Autodesk Fusion 360 part; units mm, degrees
(part 2 of 2)
sketch "Sketch4 (2)" plane through (0, -8, 0) normal (0, 1, 0) x (-1, 0, 0) in component "Middle_Cover"
  arc A0 (-84, -10) -> (-90, -16) centre (-84, -16) ccw
  line L0 (-90, -16) -> (-90, -28)
  arc A1 (-90, -28) -> (-84, -34) centre (-84, -28) ccw
  line L1 (-84, -34) -> (-16, -34)
  arc A2 (-16, -34) -> (-10, -28) centre (-16, -28) ccw
  line L2 (-10, -28) -> (-10, -16)
  arc A3 (-10, -16) -> (-16, -10) centre (-16, -16) ccw
  line L3 (-16, -10) -> (-84, -10)
  line L4 (-50, -22) -> (-90, -22) construction
  line L5 (-80, -12) -> (-60, -12) construction
  line L6 (-60, -12) -> (-60, -32) construction
  line L7 (-60, -32) -> (-80, -32) construction
  line L8 (-80, -32) -> (-80, -12) construction
  line L9 (-80, -12) -> (-60, -32) construction
  line L10 (-60, -12) -> (-80, -32) construction
  line L11 (-80, -32) -> (-60, -32) construction
  line L12 (-60, -32) -> (-60, -30) construction
  line L13 (-60, -30) -> (-80, -30) construction
  line L14 (-80, -30) -> (-80, -32) construction
  line L15 (-60, -30) -> (-80, -30) construction
  line L16 (-80, -30) -> (-80, -28) construction
  line L17 (-80, -28) -> (-60, -28) construction
  line L18 (-60, -28) -> (-60, -30) construction
  line L19 (-60, -28) -> (-80, -28) construction
  line L20 (-80, -28) -> (-80, -26) construction
  line L21 (-80, -26) -> (-60, -26) construction
  line L22 (-60, -26) -> (-60, -28) construction
  line L23 (-60, -26) -> (-80, -26) construction
  line L24 (-80, -26) -> (-80, -24) construction
  line L25 (-80, -24) -> (-60, -24) construction
  line L26 (-60, -24) -> (-60, -26) construction
  line L27 (-60, -22) -> (-80, -22) construction
  line L28 (-80, -22) -> (-80, -24) construction
  line L29 (-80, -24) -> (-60, -24) construction
  line L30 (-60, -24) -> (-60, -22) construction
  line L31 (-60, -22) -> (-80, -22) construction
  line L32 (-80, -22) -> (-80, -20) construction
  line L33 (-80, -20) -> (-60, -20) construction
  line L34 (-60, -20) -> (-60, -22) construction
  line L35 (-60, -20) -> (-80, -20) construction
  line L36 (-80, -20) -> (-80, -18) construction
  line L37 (-80, -18) -> (-60, -18) construction
  line L38 (-60, -18) -> (-60, -20) construction
  line L39 (-60, -18) -> (-80, -18) construction
  line L40 (-80, -18) -> (-80, -16) construction
  line L41 (-80, -16) -> (-60, -16) construction
  line L42 (-60, -16) -> (-60, -18) construction
  line L43 (-60, -16) -> (-80, -16) construction
  line L44 (-80, -16) -> (-80, -14) construction
  line L45 (-80, -14) -> (-60, -14) construction
  line L46 (-60, -14) -> (-60, -16) construction
  line L47 (-80, -12) -> (-78, -12) construction
  line L48 (-78, -12) -> (-78, -32) construction
  line L49 (-78, -32) -> (-80, -32) construction
  line L50 (-80, -32) -> (-80, -12) construction
  line L51 (-78, -32) -> (-76, -32) construction
  line L52 (-76, -32) -> (-76, -12) construction
  line L53 (-76, -12) -> (-78, -12) construction
  line L54 (-78, -12) -> (-78, -32) construction
  line L55 (-76, -32) -> (-74, -32) construction
  line L56 (-74, -32) -> (-74, -12) construction
  line L57 (-74, -12) -> (-76, -12) construction
  line L58 (-76, -12) -> (-76, -32) construction
  line L59 (-74, -32) -> (-72, -32) construction
  line L60 (-72, -32) -> (-72, -12) construction
  line L61 (-72, -12) -> (-74, -12) construction
  line L62 (-74, -12) -> (-74, -32) construction
  line L63 (-72, -32) -> (-70, -32) construction
  line L64 (-70, -32) -> (-70, -12) construction
  line L65 (-70, -12) -> (-72, -12) construction
  line L66 (-72, -12) -> (-72, -32) construction
  line L67 (-70, -12) -> (-68, -12) construction
  line L68 (-68, -12) -> (-68, -32) construction
  line L69 (-68, -32) -> (-70, -32) construction
  line L70 (-70, -32) -> (-70, -12) construction
  line L71 (-68, -32) -> (-66, -32) construction
  line L72 (-66, -32) -> (-66, -12) construction
  line L73 (-66, -12) -> (-68, -12) construction
  line L74 (-68, -12) -> (-68, -32) construction
  line L75 (-66, -32) -> (-64, -32) construction
  line L76 (-64, -32) -> (-64, -12) construction
  line L77 (-64, -12) -> (-66, -12) construction
  line L78 (-66, -12) -> (-66, -32) construction
  line L79 (-64, -32) -> (-62, -32) construction
  line L80 (-62, -32) -> (-62, -12) construction
  line L81 (-62, -12) -> (-64, -12) construction
  line L82 (-64, -12) -> (-64, -32) construction
  circle A4 centre (-78, -30) radius 1.5
  circle A5 centre (-78, -26) radius 1.5
  circle A6 centre (-78, -22) radius 1.5
  circle A7 centre (-78, -18) radius 1.5
  circle A8 centre (-78, -14) radius 1.5
  circle A9 centre (-74, -14) radius 1.5
  circle A10 centre (-74, -18) radius 1.5
  circle A11 centre (-74, -22) radius 1.5
  circle A12 centre (-74, -26) radius 1.5
  circle A13 centre (-74, -30) radius 1.5
  circle A14 centre (-70, -30) radius 1.5
  circle A15 centre (-70, -26) radius 1.5
  circle A16 centre (-70, -22) radius 1.5
  circle A17 centre (-70, -18) radius 1.5
  circle A18 centre (-70, -14) radius 1.5
  circle A19 centre (-66, -14) radius 1.5
  circle A20 centre (-66, -18) radius 1.5
  circle A21 centre (-66, -22) radius 1.5
  circle A22 centre (-66, -26) radius 1.5
  circle A23 centre (-66, -30) radius 1.5
  circle A24 centre (-62, -30) radius 1.5
  circle A25 centre (-62, -26) radius 1.5
  circle A26 centre (-62, -22) radius 1.5
  circle A27 centre (-62, -18) radius 1.5
  circle A28 centre (-62, -14) radius 1.5
  line L83 (-50, -22) -> (-10, -22) construction
  line L84 (-40, -12) -> (-20, -12) construction
  line L85 (-20, -12) -> (-20, -32) construction
  line L86 (-20, -32) -> (-40, -32) construction
  line L87 (-40, -32) -> (-40, -12) construction
  line L88 (-40, -12) -> (-20, -32) construction
  line L89 (-20, -12) -> (-40, -32) construction
  line L90 (-20, -12) -> (-22, -12) construction
  line L91 (-22, -12) -> (-22, -32) construction
  line L92 (-22, -32) -> (-20, -32) construction
  line L93 (-20, -32) -> (-20, -12) construction
  line L94 (-22, -32) -> (-24, -32) construction
  line L95 (-24, -32) -> (-24, -12) construction
  line L96 (-24, -12) -> (-22, -12) construction
  line L97 (-22, -12) -> (-22, -32) construction
  line L98 (-24, -12) -> (-26, -12) construction
  line L99 (-26, -12) -> (-26, -32) construction
  line L100 (-26, -32) -> (-24, -32) construction
  line L101 (-24, -32) -> (-24, -12) construction
  line L102 (-26, -32) -> (-28, -32) construction
  line L103 (-28, -32) -> (-28, -12) construction
  line L104 (-28, -12) -> (-26, -12) construction
  line L105 (-26, -12) -> (-26, -32) construction
  line L106 (-28, -12) -> (-30, -12) construction
  line L107 (-30, -12) -> (-30, -32) construction
  line L108 (-30, -32) -> (-28, -32) construction
  line L109 (-28, -32) -> (-28, -12) construction
  line L110 (-30, -32) -> (-32, -32) construction
  line L111 (-32, -32) -> (-32, -12) construction
  line L112 (-32, -12) -> (-30, -12) construction
  line L113 (-30, -12) -> (-30, -32) construction
  line L114 (-32, -12) -> (-34, -12) construction
  line L115 (-34, -12) -> (-34, -32) construction
  line L116 (-34, -32) -> (-32, -32) construction
  line L117 (-32, -32) -> (-32, -12) construction
  line L118 (-34, -32) -> (-36, -32) construction
  line L119 (-36, -32) -> (-36, -12) construction
  line L120 (-36, -12) -> (-34, -12) construction
  line L121 (-34, -12) -> (-34, -32) construction
  line L122 (-36, -12) -> (-38, -12) construction
  line L123 (-38, -12) -> (-38, -32) construction
  line L124 (-38, -32) -> (-36, -32) construction
  line L125 (-36, -32) -> (-36, -12) construction
  line L126 (-40, -12) -> (-20, -12) construction
  line L127 (-20, -12) -> (-20, -14) construction
  line L128 (-20, -14) -> (-40, -14) construction
  line L129 (-40, -14) -> (-40, -12) construction
  line L130 (-20, -14) -> (-40, -14) construction
  line L131 (-40, -14) -> (-40, -16) construction
  line L132 (-40, -16) -> (-20, -16) construction
  line L133 (-20, -16) -> (-20, -14) construction
  line L134 (-20, -16) -> (-40, -16) construction
  line L135 (-40, -16) -> (-40, -18) construction
  line L136 (-40, -18) -> (-20, -18) construction
  line L137 (-20, -18) -> (-20, -16) construction
  line L138 (-40, -18) -> (-20, -18) construction
  line L139 (-20, -18) -> (-20, -20) construction
  line L140 (-20, -20) -> (-40, -20) construction
  line L141 (-40, -20) -> (-40, -18) construction
  line L142 (-40, -22) -> (-20, -22) construction
  line L143 (-20, -22) -> (-20, -24) construction
  line L144 (-20, -24) -> (-40, -24) construction
  line L145 (-40, -24) -> (-40, -22) construction
  line L146 (-40, -24) -> (-20, -24) construction
  line L147 (-20, -24) -> (-20, -26) construction
  line L148 (-20, -26) -> (-40, -26) construction
  line L149 (-40, -26) -> (-40, -24) construction
  line L150 (-40, -26) -> (-20, -26) construction
  line L151 (-20, -26) -> (-20, -28) construction
  line L152 (-20, -28) -> (-40, -28) construction
  line L153 (-40, -28) -> (-40, -26) construction
  line L154 (-40, -28) -> (-20, -28) construction
  line L155 (-20, -28) -> (-20, -30) construction
  line L156 (-20, -30) -> (-40, -30) construction
  line L157 (-40, -30) -> (-40, -28) construction
  circle A29 centre (-38, -30) radius 1.5
  circle A30 centre (-38, -26) radius 1.5
  circle A31 centre (-38, -22) radius 1.5
  circle A32 centre (-38, -18) radius 1.5
  circle A33 centre (-38, -14) radius 1.5
  circle A34 centre (-34, -14) radius 1.5
  circle A35 centre (-34, -18) radius 1.5
  circle A36 centre (-34, -22) radius 1.5
  circle A37 centre (-34, -26) radius 1.5
  circle A38 centre (-34, -30) radius 1.5
  circle A39 centre (-30, -30) radius 1.5
  circle A40 centre (-30, -26) radius 1.5
  circle A41 centre (-30, -22) radius 1.5
  circle A42 centre (-30, -18) radius 1.5
  circle A43 centre (-30, -14) radius 1.5
  circle A44 centre (-26, -14) radius 1.5
  circle A45 centre (-22, -14) radius 1.5
  circle A46 centre (-26, -18) radius 1.5
  circle A47 centre (-22, -18) radius 1.5
  circle A48 centre (-26, -22) radius 1.5
  circle A49 centre (-22, -22) radius 1.5
  circle A50 centre (-26, -26) radius 1.5
  circle A51 centre (-22, -26) radius 1.5
  circle A52 centre (-22, -30) radius 1.5
  circle A53 centre (-26, -30) radius 1.5
  point P0 (-70, -22)
  point P1 (-30, -22)
  dimension "d20_1" = 20
  dimension "d21_1" = 20
  dimension "d22_1" = 2
  dimension "d23_1" = 2
  dimension "d24_1" = 2
  dimension "d25_1" = 2
  dimension "d26_1" = 2
  dimension "d27_1" = 2
  dimension "d28_1" = 2
  dimension "d29_1" = 2
  dimension "d30_1" = 2
  dimension "d31_1" = 2
  dimension "d32_1" = 2
  dimension "d33_1" = 2
  dimension "d34_1" = 2
  dimension "d35_1" = 3
  dimension "d36_1" = 3
  dimension "d37_1" = 3
  dimension "d38_1" = 3
  dimension "d39_1" = 3
  dimension "d40_1" = 3
  dimension "d41_1" = 3
  dimension "d42_1" = 3
  dimension "d43_1" = 3
  dimension "d44_1" = 3
  dimension "d45_1" = 3
  dimension "d46_1" = 3
  dimension "d47_1" = 3
  dimension "d48_1" = 3
  dimension "d49_1" = 3
  dimension "d50_1" = 3
  dimension "d51_1" = 3
  dimension "d52_1" = 3
  dimension "d53_1" = 3
  dimension "d54_1" = 3
  dimension "d55_1" = 3
  dimension "d56_1" = 3
  dimension "d57_1" = 3
  dimension "d58_1" = 3
  dimension "d59_1" = 3
  dimension "d62_1" = 20
  dimension "d63_1" = 20
  dimension "d64_1" = 2
  dimension "d65_1" = 20
  dimension "d66_1" = 2
  dimension "d67_1" = 2
  dimension "d68_1" = 2
  dimension "d69_1" = 2
  dimension "d70_1" = 2
  dimension "d71_1" = 20
  dimension "d72_1" = 2
  dimension "d73_1" = 2
  dimension "d74_1" = 2
  dimension "d75_1" = 2
  dimension "d76_1" = 2
  dimension "d77_1" = 2
  dimension "d78_1" = 3
  dimension "d79_1" = 3
  dimension "d80_1" = 3
  dimension "d81_1" = 3
  dimension "d82_1" = 3
  dimension "d83_1" = 3
  dimension "d84_1" = 3
  dimension "d85_1" = 3
  dimension "d86_1" = 3
  dimension "d87_1" = 3
  dimension "d88_1" = 3
  dimension "d89_1" = 3
  dimension "d90_1" = 3
  dimension "d91_1" = 3
  dimension "d92_1" = 3
  dimension "d93_1" = 3
  dimension "d94_1" = 3
  dimension "d95_1" = 3
  dimension "d96_1" = 3
  dimension "d97_1" = 3
  dimension "d98_1" = 3
  dimension "d99_1" = 3
  dimension "d100_1" = 3
  dimension "d101_1" = 3
  dimension "d102_1" = 3
  constraint midpoint L0 L4.end
  constraint perpendicular L5 L6
  constraint parallel L5 L7
  constraint parallel L6 L8
  constraint horizontal L5
  constraint coincident L9 P0
  constraint coincident L10 P0
  constraint midpoint L4 P0
  constraint horizontal L11
  constraint vertical L12
  constraint horizontal L13
  constraint vertical L14
  constraint horizontal L15
  constraint vertical L16
  constraint horizontal L17
  constraint vertical L18
  constraint horizontal L19
  constraint vertical L20
  constraint horizontal L21
  constraint vertical L22
  constraint horizontal L23
  constraint vertical L24
  constraint horizontal L25
  constraint vertical L26
  constraint horizontal L27
  constraint vertical L28
  constraint horizontal L29
  constraint vertical L30
  constraint midpoint L6 L27.start
  constraint horizontal L31
  constraint vertical L32
  constraint horizontal L33
  constraint vertical L34
  constraint coincident L8 L32.end
  constraint horizontal L35
  constraint vertical L36
  constraint horizontal L37
  constraint vertical L38
  constraint coincident L8 L36.end
  constraint horizontal L39
  constraint vertical L40
  constraint horizontal L41
  constraint vertical L42
  constraint horizontal L43
  constraint vertical L44
  constraint horizontal L45
  constraint vertical L46
  constraint horizontal L47
  constraint vertical L48
  constraint horizontal L49
  constraint vertical L50
  constraint horizontal L51
  constraint vertical L52
  constraint horizontal L53
  constraint vertical L54
  constraint horizontal L55
  constraint vertical L56
  constraint horizontal L57
  constraint vertical L58
  constraint horizontal L59
  constraint vertical L60
  constraint horizontal L61
  constraint vertical L62
  constraint horizontal L63
  constraint vertical L64
  constraint horizontal L65
  constraint vertical L66
  constraint horizontal L67
  constraint vertical L68
  constraint horizontal L69
  constraint vertical L70
  constraint horizontal L71
  constraint vertical L72
  constraint horizontal L73
  constraint vertical L74
  constraint horizontal L75
  constraint vertical L76
  constraint horizontal L77
  constraint vertical L78
  constraint horizontal L79
  constraint vertical L80
  constraint horizontal L81
  constraint vertical L82
  constraint coincident L48 A4.centre
  constraint coincident L13 A4.centre
  constraint coincident L48 A5.centre
  constraint coincident L23 A5.centre
  constraint midpoint L48 A6.centre
  constraint coincident L54 A7.centre
  constraint coincident L37 A7.centre
  constraint coincident L48 A8.centre
  constraint coincident L45 A8.centre
  constraint coincident L56 A9.centre
  constraint coincident L45 A9.centre
  constraint coincident L56 A10.centre
  constraint coincident L39 A10.centre
  constraint midpoint L62 A11.centre
  constraint coincident L62 A12.centre
  constraint coincident L21 A12.centre
  constraint coincident L56 A13.centre
  constraint coincident L13 A13.centre
  constraint midpoint L13 A14.centre
  constraint midpoint L21 A15.centre
  constraint coincident P0 A16.centre
  constraint midpoint L39 A17.centre
  constraint midpoint L45 A18.centre
  constraint coincident L72 A19.centre
  constraint coincident L45 A19.centre
  constraint coincident L72 A20.centre
  constraint coincident L39 A20.centre
  constraint midpoint L72 A21.centre
  constraint coincident L72 A22.centre
  constraint coincident L21 A22.centre
  constraint coincident L78 A23.centre
  constraint coincident L15 A23.centre
  constraint coincident L80 A24.centre
  constraint coincident L15 A24.centre
  constraint coincident L80 A25.centre
  constraint coincident L23 A25.centre
  constraint midpoint L80 A26.centre
  constraint coincident L80 A27.centre
  constraint coincident L37 A27.centre
  constraint coincident L80 A28.centre
  constraint coincident L10 A28.centre
  constraint midpoint L2 L83.end
  constraint perpendicular L84 L85
  constraint parallel L84 L86
  constraint parallel L85 L87
  constraint horizontal L84
  constraint coincident L88 P1
  constraint coincident L89 P1
  constraint midpoint L83 P1
  constraint horizontal L90
  constraint vertical L91
  constraint horizontal L92
  constraint vertical L93
  constraint coincident L86 L91.end
  constraint horizontal L94
  constraint vertical L95
  constraint horizontal L96
  constraint vertical L97
  constraint coincident L84 L95.end
  constraint horizontal L98
  constraint vertical L99
  constraint horizontal L100
  constraint vertical L101
  constraint coincident L86 L99.end
  constraint horizontal L102
  constraint vertical L103
  constraint horizontal L104
  constraint vertical L105
  constraint horizontal L106
  constraint vertical L107
  constraint horizontal L108
  constraint vertical L109
  constraint midpoint L86 L107.end
  constraint horizontal L110
  constraint vertical L111
  constraint horizontal L112
  constraint vertical L113
  constraint coincident L84 L111.end
  constraint horizontal L114
  constraint vertical L115
  constraint horizontal L116
  constraint vertical L117
  constraint coincident L86 L115.end
  constraint horizontal L118
  constraint vertical L119
  constraint horizontal L120
  constraint vertical L121
  constraint horizontal L122
  constraint vertical L123
  constraint horizontal L124
  constraint vertical L125
  constraint horizontal L126
  constraint vertical L127
  constraint horizontal L128
  constraint vertical L129
  constraint horizontal L130
  constraint vertical L131
  constraint horizontal L132
  constraint vertical L133
  constraint horizontal L134
  constraint vertical L135
  constraint horizontal L136
  constraint vertical L137
  constraint horizontal L138
  constraint vertical L139
  constraint horizontal L140
  constraint vertical L141
  constraint horizontal L142
  constraint vertical L143
  constraint horizontal L144
  constraint vertical L145
  constraint midpoint L87 L142.start
  constraint horizontal L146
  constraint vertical L147
  constraint horizontal L148
  constraint vertical L149
  constraint horizontal L150
  constraint vertical L151
  constraint horizontal L152
  constraint vertical L153
  constraint horizontal L154
  constraint vertical L155
  constraint horizontal L156
  constraint vertical L157
  constraint coincident L123 A29.centre
  constraint coincident L156 A29.centre
  constraint coincident L148 A30.centre
  constraint coincident L123 A30.centre
  constraint midpoint L123 A31.centre
  constraint coincident L123 A32.centre
  constraint coincident L136 A32.centre
  constraint coincident L88 A33.centre
  constraint coincident L128 A33.centre
  constraint coincident L121 A34.centre
  constraint coincident L128 A34.centre
  constraint coincident L136 A35.centre
  constraint coincident L115 A35.centre
  constraint midpoint L115 A36.centre
  constraint coincident L121 A37.centre
  constraint coincident L150 A37.centre
  constraint coincident L121 A38.centre
  constraint coincident L156 A38.centre
  constraint midpoint L156 A39.centre
  constraint midpoint L148 A40.centre
  constraint coincident P1 A41.centre
  constraint midpoint L136 A42.centre
  constraint midpoint L128 A43.centre
  constraint coincident L105 A44.centre
  constraint coincident L130 A44.centre
  constraint coincident L128 A45.centre
  constraint coincident L89 A45.centre
  constraint coincident L138 A46.centre
  constraint coincident L89 A46.centre
  constraint coincident L91 A47.centre
  constraint coincident L136 A47.centre
  constraint midpoint L105 A48.centre
  constraint midpoint L91 A49.centre
  constraint coincident L99 A50.centre
  constraint coincident L148 A50.centre
  constraint coincident L148 A51.centre
  constraint coincident L91 A51.centre
  constraint coincident L97 A52.centre
  constraint coincident L156 A52.centre
  constraint coincident L99 A53.centre
  constraint coincident L156 A53.centre
  measures "d20_1" distance of L6.end L7.end
  measures "d21_1" distance of L5.end L6.end
  measures "d22_1" distance of L7.end L13.end
  measures "d23_1" distance of L12.end L17.end
  measures "d24_1" distance of L17.end L21.end
  measures "d25_1" distance of L21.end L25.end
  measures "d26_1" distance of L5.start L47.end
  measures "d27_1" distance of L48.end L51.end
  measures "d28_1" distance of L51.end L55.end
  measures "d29_1" distance of L55.end L59.end
  measures "d30_1" distance of L59.end L63.end
  measures "d31_1" distance of L64.end L67.end
  measures "d32_1" distance of L68.end L71.end
  measures "d33_1" distance of L71.end L75.end
  measures "d34_1" distance of L75.end L79.end
  measures "d35_1" diameter of A4
  measures "d36_1" diameter of A5
  measures "d37_1" diameter of A6
  measures "d38_1" diameter of A7
  measures "d39_1" diameter of A8
  measures "d40_1" diameter of A9
  measures "d41_1" diameter of A10
  measures "d42_1" diameter of A11
  measures "d43_1" diameter of A12
  measures "d44_1" diameter of A13
  measures "d45_1" diameter of A14
  measures "d46_1" diameter of A15
  measures "d47_1" diameter of A16
  measures "d48_1" diameter of A17
  measures "d49_1" diameter of A18
  measures "d50_1" diameter of A19
  measures "d51_1" diameter of A20
  measures "d52_1" diameter of A21
  measures "d53_1" diameter of A22
  measures "d54_1" diameter of A23
  measures "d55_1" diameter of A24
  measures "d56_1" diameter of A25
  measures "d57_1" diameter of A26
  measures "d58_1" diameter of A27
  measures "d59_1" diameter of A28
  measures "d62_1" distance of L85.end L86.end
  measures "d63_1" distance of L84.end L85.end
  measures "d64_1" distance of L95.end L98.end
  measures "d65_1" distance of L99.end L98.end
  measures "d66_1" distance of L99.end L102.end
  measures "d67_1" distance of L115.end L118.end
  measures "d68_1" distance of L119.end L122.end
  measures "d69_1" distance of L84.start L128.end
  measures "d70_1" distance of L127.end L132.end
  measures "d71_1" distance of L132.end L131.end
  measures "d72_1" distance of L132.end L136.end
  measures "d73_1" distance of L135.end L140.end
  measures "d74_1" distance of L142.start L144.end
  measures "d75_1" distance of L144.end L148.end
  measures "d76_1" distance of L148.end L152.end
  measures "d77_1" distance of L152.end L156.end
  measures "d78_1" diameter of A29
  measures "d79_1" diameter of A30
  measures "d80_1" diameter of A31
  measures "d81_1" diameter of A32
  measures "d82_1" diameter of A33
  measures "d83_1" diameter of A34
  measures "d84_1" diameter of A35
  measures "d85_1" diameter of A36
  measures "d86_1" diameter of A37
  measures "d87_1" diameter of A38
  measures "d88_1" diameter of A39
  measures "d89_1" diameter of A40
  measures "d90_1" diameter of A41
  measures "d91_1" diameter of A42
  measures "d92_1" diameter of A43
  measures "d93_1" diameter of A44
  measures "d94_1" diameter of A45
  measures "d95_1" diameter of A46
  measures "d96_1" diameter of A47
  measures "d97_1" diameter of A48
  measures "d98_1" diameter of A49
  measures "d99_1" diameter of A50
  measures "d100_1" diameter of A51
  measures "d101_1" diameter of A52
  measures "d102_1" diameter of A53
extrude "Extrude5'" cut sketch "Sketch4 (2)" against normal up to surface (3 mm away) contours A29 | A30 | A31 | A32 | A33 | A34 | A35 | A36 | A37 | A38 | A39 | A40 | A41 | A42 | A43 | A44 | A45 | A46 | A47 | A48 | A49 | A50 | A51 | A52 | A53 bodies 3 in component "Middle_Cover"
extrude "Extrude4'" cut sketch "Sketch4 (2)" against normal up to surface (3 mm away) contours A4 | A5 | A6 | A7 | A8 | A9 | A10 | A11 | A12 | A13 | A14 | A15 | A16 | A17 | A18 | A19 | A20 | A21 | A22 | A23 | A24 | A25 | A26 | A27 | A28 bodies 3 in component "Middle_Cover"
sketch "Sketch5 (2)" plane through (0, 0, 0) normal (0, 1, 0) x (-1, 0, 0) in component "Middle_Cover"
  circle A0 centre (-85, -39) radius 1.95
  circle A1 centre (-15, -39) radius 1.95
  circle A2 centre (-85, -5) radius 1.95
  circle A3 centre (-15, -5) radius 1.95
  line L0 (-16, -34) -> (-84, -34)
  arc A4 (-90, -28) -> (-84, -34) centre (-84, -28) ccw
  line L1 (-90, -28) -> (-90, -16)
  arc A5 (-84, -10) -> (-90, -16) centre (-84, -16) ccw
  line L2 (-84, -10) -> (-16, -10)
  arc A6 (-10, -16) -> (-16, -10) centre (-16, -16) ccw
  line L3 (-10, -16) -> (-10, -28)
  arc A7 (-16, -34) -> (-10, -28) centre (-16, -28) ccw
  arc A8 (-94, 0) -> (-100, -6) centre (-94, -6) ccw
  line L4 (-100, -6) -> (-100, -38)
  arc A9 (-100, -38) -> (-94, -44) centre (-94, -38) ccw
  line L5 (-94, -44) -> (-6, -44)
  arc A10 (-6, -44) -> (0, -38) centre (-6, -38) ccw
  line L6 (0, -38) -> (0, -6)
  arc A11 (0, -6) -> (-6, 0) centre (-6, -6) ccw
  line L7 (-6, 0) -> (-94, 0)
  line L8 (0, -22) -> (0, -25) construction
  line L9 (0, -25) -> (-10, -25)
  line L10 (-10, -25) -> (-10, -19)
  line L11 (-10, -19) -> (0, -19)
  line L12 (0, -19) -> (0, -25)
  dimension "d105_1" = 3
  dimension "d106_1" = 6
  constraint midpoint L6 L8.start
  constraint parallel L6 L8
  constraint horizontal L9
  constraint vertical L10
  constraint horizontal L11
  constraint vertical L12
  measures "d105_1" distance of L8.start L8.end
  measures "d106_1" distance of L8.end L11.end
extrude "Extrude6'" cut sketch "Sketch5 (2)" against normal blind 3 contours L3 L6 L9 L10 L11 L12 bodies 3 in component "Middle_Cover"
sketch "Sketch6 (2)" plane through (0, 0, 0) normal (0, 1, 0) x (1, 0, 0) in component "Middle_Cover"
  line L0 (100, 22) -> (100, 24.5) construction
  line L1 (100, 24.5) -> (90, 24.5)
  line L2 (90, 24.5) -> (90, 19.5)
  line L3 (90, 19.5) -> (100, 19.5)
  line L4 (100, 19.5) -> (100, 24.5)
  dimension "d109_1" = 2.5
  dimension "d110_1" = 5
  constraint vertical L0
  constraint horizontal L1
  constraint vertical L2
  constraint horizontal L3
  constraint vertical L4
  measures "d109_1" distance of L0.start L0.end
  measures "d110_1" distance of L0.end L3.end
extrude "Extrude7'" cut sketch "Sketch6 (2)" against normal blind 2.5 bodies 3 in component "Middle_Cover"
move_face "MoveFace1" by (0, -4, 0) 1 faces at (13.5, -8, -22) on bodies 3 in component "Middle_Cover"
delete_face "DeleteFace1" 1 faces at (98.7163, -3.6667, -2.291) on bodies 3 in component "Middle_Cover"
fillet "Fillet2" radius 6 1 edges at (100, -5.5, 0) on bodies 3 in component "Middle_Cover"
move_face "OffsetFaces1" offset 1 1 faces at (64.6667, -11, -14.6667) on bodies 1 in component "Bottom_Cover"
move_face "OffsetFaces1'" offset 1 1 faces at (6.8333, -11, -22) on bodies 2 in component "Top_Cover"
move_face "OffsetFaces1''" offset 1 1 faces at (3.3333, -11, -24) on bodies 3 in component "Middle_Cover"
sketch "Sketch1 (4)" plane through (0, 0, 0) normal (0, 1, 0) x (1, 0, 0) in component "All_Covers"
  line L0 (0, 0) -> (100, 0)
  line L1 (100, 0) -> (100, 44)
  line L2 (100, 44) -> (0, 44)
  line L3 (0, 44) -> (0, 0)
  line L4 (0, 22) -> (100, 22) construction
  line L5 (50, 44) -> (50, 0) construction
  line L6 (90, 10) -> (10, 10)
  line L7 (10, 10) -> (10, 34)
  line L8 (10, 34) -> (90, 34)
  line L9 (90, 34) -> (90, 10)
  line L10 (90, 10) -> (10, 34) construction
  line L11 (10, 10) -> (90, 34) construction
  point P0 (50, 22)
  dimension "d1_2" = 100
  dimension "d2_2" = 44
  dimension "d3_2" = 80
  dimension "d4_2" = 24
  constraint horizontal L0
  constraint vertical L1
  constraint horizontal L2
  constraint vertical L3
  constraint coincident L0.start L3.end
  constraint midpoint L3 L4.start
  constraint midpoint L1 L4.end
  constraint midpoint L2 L5.start
  constraint midpoint L0 L5.end
  constraint perpendicular L6 L7
  constraint parallel L6 L8
  constraint parallel L7 L9
  constraint horizontal L6
  constraint coincident L10 P0
  constraint coincident L11 P0
  constraint midpoint L4 P0
  measures "d1_2" distance of L0.start L0.end
  measures "d2_2" distance of L0.start L2.end
  measures "d3_2" distance of L7.end L8.end
  measures "d4_2" distance of L6.end L7.end
extrude "Extrude1'''" add sketch "Sketch1 (4)" against normal blind 11 separate body makes body 4 in component "All_Covers"
sketch "Sketch2 (4)" plane through (0, -11, 0) normal (0, -1, 0) x (1, 0, 0) in component "All_Covers"
  line L0 (90, -34) -> (10, -34)
  line L1 (10, -34) -> (10, -10)
  line L2 (10, -10) -> (90, -10)
  line L3 (90, -10) -> (90, -34)
  line L4 (0, 0) -> (0, -44)
  line L5 (0, -44) -> (100, -44)
  line L6 (100, -44) -> (100, 0)
  line L7 (100, 0) -> (0, 0)
  line L8 (10, -10) -> (90, -10)
  line L9 (90, -10) -> (90, -34)
  line L10 (90, -34) -> (10, -34)
  line L11 (10, -34) -> (10, -10)
  constraint horizontal L8
  constraint vertical L9
  constraint horizontal L10
  constraint vertical L11
  constraint coincident L0.start L3.end
  constraint coincident L1.end L2.start
extrude "Extrude2'''" add sketch "Sketch2 (4)" against normal blind 3 contours L0 L1 L2 L3 L8 L9 L10 L11 bodies 4 in component "All_Covers"
fillet "Fillet1'''" radius 6 8 edges at (10, -4, -34) (10, -4, -10) (90, -4, -34) (90, -4, -10) (100, -5.5, -44) (0, -5.5, -44) (0, -5.5, 0) (100, -5.5, 0) on bodies 4 in component "All_Covers"
sketch "Sketch3 (4)" plane through (0, 0, 0) normal (0, 1, 0) x (1, 0, 0) in component "All_Covers"
  line L0 (50, 34) -> (50, 44) construction
  line L1 (50, 39) -> (100, 39) construction
  line L2 (100, 39) -> (50, 39) construction
  line L3 (50, 39) -> (0, 39) construction
  line L4 (50, 10) -> (50, 0) construction
  line L5 (50, 0) -> (50, 5) construction
  line L6 (100, 5) -> (50, 5) construction
  line L7 (50, 5) -> (0, 5) construction
  line L8 (50, 39) -> (85, 39) construction
  line L9 (50, 5) -> (85, 5) construction
  line L10 (50, 5) -> (15, 5) construction
  line L11 (50, 39) -> (15, 39) construction
  circle A0 centre (85, 5) radius 1.95
  circle A1 centre (85, 39) radius 1.95
  circle A2 centre (15, 39) radius 1.95
  circle A3 centre (15, 5) radius 1.95
  point P0 (85, 39)
  point P1 (85, 5)
  point P2 (15, 5)
  point P3 (15, 39)
  dimension "d10_2" = 35
  dimension "d11_2" = 35
  dimension "d12_2" = 35
  dimension "d13_2" = 35
  dimension "d14_2" = 3.9
  dimension "d15_2" = 3.9
  dimension "d16_2" = 3.9
  dimension "d17_2" = 3.9
  constraint vertical L0
  constraint midpoint L0 L1.start
  constraint perpendicular L0 L1
  constraint perpendicular L0 L3
  constraint vertical L4
  constraint midpoint L4 L5.end
  constraint perpendicular L4 L6
  constraint perpendicular L5 L7
  constraint perpendicular L0 L8
  constraint perpendicular L5 L9
  constraint perpendicular L4 L10
  constraint parallel L3 L11
  constraint coincident P0 L8.end
  constraint coincident P1 L9.end
  constraint coincident P2 L10.end
  constraint coincident P3 L11.end
  measures "d10_2" distance of L1.start P0
  measures "d11_2" distance of L5.end P1
  measures "d12_2" distance of L5.end P2
  measures "d13_2" distance of L1.start L11.end
  measures "d14_2" diameter of A0
  measures "d15_2" diameter of A1
  measures "d16_2" diameter of A2
  measures "d17_2" diameter of A3
extrude "Extrude3'''" cut sketch "Sketch3 (4)" against normal blind 5 bodies 4 in component "All_Covers"
move_face "OffsetFaces1'''" offset 1 1 faces at (64.6667, -11, -14.6667) on bodies 4 in component "All_Covers"
copy_body "CopyPasteBodies1" bodies 2 body 2 seen with x (1, 0, 0) y (0, 1, 0) z (0, 0, 1) at (0, 0, -59) makes body 5 in component "All_Covers"
copy_body "CopyPasteBodies2" bodies 3 body 3 seen with x (1, 0, 0) y (0, 1, 0) z (0, 0, 1) at (0, 0, -118) makes body 6 in component "All_Covers"
component "Bottom_Cover" placed x (1, 0, 0) y (0, 1, 0) z (0, 0, 1) at (0, 12, 0)
component "Top_Cover" placed x (1, 0, 0) y (0, 1, 0) z (0, 0, 1) at (0, 12, -59)
component "Middle_Cover" placed x (1, 0, 0) y (0, 1, 0) z (0, 0, 1) at (0, 12, -118)
component "All_Covers" placed x (1, 0, 0) y (0, 1, 0) z (0, 0, 1) at (0, 12, 0)
named bodies: "Bottom", "Top"
